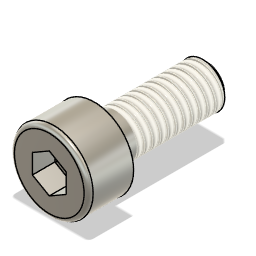
EchoWeather_WindVane (Autodesk Fusion 360 archive; units mm, degrees)
design "Broached Hexagon Socket Head Cap Screw ASME B18.3.1M - M4x0.7 x 10 Steel Grade 2 Plain"
description: Broached Hexagon Socket Head Cap Screw ASME B18.3.1M - M4x0.7 x 10
part number: BSHCS ASME B18.3.1M - M4x0.7 x 10 Steel Grade 2 Plain
Autodesk Fusion 360 part; units mm, degrees
note: some values were not read from the file. Chosen so that the rebuilt part matches the saved one: which bodies a step acts on; how an offset face is resized. Set by a fixed rule: which sketch regions a step uses.
sketch "Sketch1" plane through (0, 0, 0) normal (0, 1, 0) x (1, 0, 0)
  line L0 (-2, 0) -> (-2, 10)
  line L1 (-2, 10) -> (0, 10)
  line L2 (0, 10) -> (0, -4)
  line L3 (-2, 0) -> (-3.5, 0)
  line L4 (-3.5, 0) -> (-3.5, -4)
  line L5 (-3.5, -4) -> (0, -4)
  dimension "d9" = 4
  dimension "d66" = 7
  dimension "d101" = 10
  dimension "d102" = 4
  constraint perpendicular L0 L1
  constraint collinear origin L1.end L2.end
  constraint perpendicular L0 L3
  constraint coincident origin L3
  constraint vertical L0
  constraint vertical L2
  constraint parallel L2 L4
  constraint coincident L2 L5.end
  constraint perpendicular L2 L5
  measures "d101" distance of origin L1
  measures "d102" distance of L3.end L5
revolve "Revolve1" add sketch "Sketch1" angle 360 about axis through (0, 0, -10) along (0, 0, 1)
ref_plane "WorkPlane1" through (0, 0, 4) normal (0, 0, 1) x (1, 0, 0)
sketch "Sketch6" plane through (0, 0, 4) normal (0, 0, 1) x (1, 0, 0)
  line L0 (-1.5, 0) -> (1.5, 0) construction
  line L1 (0, 0) -> (-1.5, 0.866)
  line L2 (-1.5, -0.866) -> (-1.5, 0.866)
  line L3 (-1.5, -0.866) -> (0, 0)
  dimension "d100" = 150
  dimension "d103" = 3
  constraint horizontal L0
  constraint midpoint L1.start L0
  constraint coincident L1.start L3.end
  constraint perpendicular L0 L2
  constraint midpoint L0.start L2
  constraint coincident L1.end L2.end
  measures "d100" angle of L0 L1
  measures "d103" distance of L0.end L2
extrude "Extrude1" cut sketch "Sketch6" against normal blind 2
pattern_circular "C-Pattern1" count 6 over 360 about axis through (0, 0, 1.75) along (0, 0, 1) of "Extrude1"
extrude "Extrude2" cut 1 faces at (0, -0.5774, 2) along direction (0, 0, -1) blind 2 draft -85
thread "Thread3" "ANSI Metric M Profile 4.0 M4x0.7 M4x0.7 4g6g" major diameter 3.908 minor diameter 3.128 pitch 0.7 angle 60 resizes the face on face at (-1.9901, 0.1991, -3.3333)
fillet "Fillet4" radius 0.4 1 edges at (-3.2631, 1.2657, 4)
sketch "Sketch7" plane through (0, 0, 0) normal (0, 1, 0) x (1, 0, 0)
  line L0 (-2.04, 10) -> (-2.04, 9.5706)
  line L1 (-2.04, 9.5706) -> (-1.5706, 10)
  line L2 (0, 10) -> (0, -4)
  line L3 (-2.04, 10) -> (0, 10)
  dimension "d104" = 1.5706
  dimension "d105" = 2.04
  dimension "d106" = 0.4294
  constraint coincident L2.start L3.end
  constraint perpendicular L2 L3
  constraint coincident L1.end L3
  constraint perpendicular L0 L3
  measures "d104" distance of L1.end L2
  measures "d105" distance of L0 L2.start
  measures "d106" distance of L0.end L3
revolve "Revolve3" cut sketch "Sketch7" angle 360 about axis through (0, 0, 1.75) along (0, 0, 1)
equation "d9 = adsk_nomdia"
equation "adsk_nomlen = 10.00 mm"
equation "adsk_headh = 4.00 mm"
equation "adsk_headdia = 7.00 mm"
equation "adsk_nomdia = 4.00 mm"
equation "adsk_philwidth = 3.00 mm"
equation "d31 = -adsk_phildepth"
equation "adsk_phildepth = 2.00 mm"
equation "d66 = adsk_headdia"
equation "d71 = adsk_headh"
equation "d76 = -adsk_phildepth"
equation "adsk_thrlen = 8.170585 mm"
equation "d86 = adsk_nomdia * 0.1"
equation "adsk_startlen = 0.429415 mm"
equation "adsk_endpointdia = 3.14117 mm"
equation "d101 = adsk_nomlen"
equation "d102 = adsk_headh"
equation "d103 = adsk_philwidth"
equation "d104 = adsk_endpointdia / 2"
equation "d105 = adsk_nomdia * 0.51"
equation "d106 = adsk_startlen"
equation "d108 = min(adsk_thrlen; adsk_nomlen - 0.001 mm)"

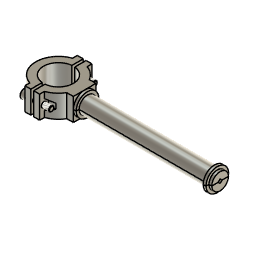
design "EchoWeather_SupportRod" references "Broached Hexagon Socket Head Cap Screw ASME B18.3.1M - M6x1 x 25 Steel Grade 2 Plain"
Autodesk Fusion 360 part; units mm, degrees
sketch "Sketch1" plane through (0, 0, 0) normal (0, 0, 1) x (1, 0, 0)
  circle A0 centre (0, 0) radius 16.764
  circle A1 centre (0, 0) radius 25.4
  dimension "d1" = 33.528
  dimension "d2" = 50.8
  constraint coincident A0.centre A1.centre
  measures "d1" diameter of A0
  measures "d2" diameter of A1
extrude "Extrude1" add sketch "Sketch1" along normal blind 25.4 makes body 1
sketch "Sketch2" plane through (0, 0, 0) normal (1, 0, 0) x (0, 1, 0)
  line L0 (0, 0) -> (0, 25.4) construction
  line L1 (25.4, 25.4) -> (-25.4, 25.4) construction
  circle A0 centre (0, 12.7) radius 9.525 construction
  line L2 (-12.7, 25.4) -> (12.7, 25.4)
  line L3 (12.7, 25.4) -> (12.7, 0)
  line L4 (12.7, 0) -> (-12.7, 0)
  line L5 (-12.7, 0) -> (-12.7, 25.4)
  line L6 (25.4, 0) -> (-25.4, 0)
  circle A1 centre (0, 12.7) radius 9.779
  dimension "d5" = 19.05
  dimension "d6" = 12.7
  dimension "d7" = 12.7
  dimension "d8" = 0.254
  constraint coincident L0.start origin
  constraint vertical L0
  constraint midpoint L0.end L1
  constraint midpoint L0 A0.centre
  constraint horizontal L2
  constraint vertical L3
  constraint horizontal L4
  constraint vertical L5
  constraint coincident L1 L2.start
  constraint coincident L3.end L6
  constraint concentric A0 A1
  measures "d5" diameter of A0
  measures "d6" distance of L0 L5
  measures "d7" distance of L0 L3
  measures "d8" distance of A0 A1
extrude "Extrude2" cut sketch "Sketch2" along normal blind 39.6494 contours A1 bodies 1
extrude "Extrude3" add sketch "Sketch2" along normal blind 12.7 from surface at 16.764 bodies 1
sketch "Sketch3" plane through (0, 0, 25.4) normal (0, 0, 1) x (-1, 0, 0)
  arc A0 (-21.997, -12.7) -> (-21.997, 12.7) centre (0, 0) ccw
  line L0 (-21.997, 12.7) -> (-29.464, 12.7)
  line L1 (-29.464, 12.7) -> (-29.464, -12.7)
  line L2 (-29.464, -12.7) -> (-21.997, -12.7)
  circle A1 centre (0, 0) radius 16.764
  line L3 (0, 0) -> (0, 34.343) construction
  line L4 (-8.255, 29.464) -> (8.255, 29.464)
  line L5 (8.255, 29.464) -> (8.255, 16.764)
  line L6 (8.255, 16.764) -> (-8.255, 16.764)
  line L7 (-8.255, 16.764) -> (-8.255, 29.464)
  line L8 (0, 0) -> (42.1929, 0) construction
  line L9 (8.255, -29.464) -> (8.255, -16.764)
  line L10 (-8.255, -16.764) -> (-8.255, -29.464)
  line L11 (-8.255, -29.464) -> (8.255, -29.464)
  line L12 (8.255, -16.764) -> (-8.255, -16.764)
  point P0 (0, -34.343)
  dimension "d14" = 12.7
  dimension "d15" = 8.255
  constraint coincident A0.centre A1.centre
  constraint parallel L1 L3
  constraint horizontal L4
  constraint vertical L5
  constraint horizontal L6
  constraint vertical L7
  constraint symmetric L3 L5 L7
  constraint tangent A1 L6
  constraint perpendicular L3 L8
  constraint symmetric L3.end L8 P0
  constraint symmetric L4.start L8 L10.end
  constraint symmetric L4.end L8 L9.start
  constraint symmetric L5.end L8 L9.end
  constraint symmetric L6.end L8 L10.start
  measures "d14" distance of L4 L6
  measures "d15" distance of L3 L5
extrude "Extrude4" add sketch "Sketch3" against normal up to surface (25.4 mm away) contours A0 L9 L10 L11 | A0 L4 L5 L7 bodies 1
sketch "Sketch4" plane through (-8.255, 0, 0) normal (-1, 0, 0) x (0, -1, 0)
  line L0 (-29.464, 0) -> (-24.0211, 0)
  line L1 (-24.0211, 0) -> (-24.0211, 25.4)
  line L2 (-24.0211, 25.4) -> (-29.464, 25.4)
  line L3 (-29.464, 25.4) -> (-29.464, 0)
  line L4 (-29.464, 12.7) -> (29.464, 12.7) construction
  line L5 (29.464, 25.4) -> (29.464, 0) construction
  circle A0 centre (-24.384, 12.7) radius 3.1
  circle A1 centre (24.384, 12.7) radius 3.1
  dimension "d18" = 6.2
  dimension "d19" = 6.2
  dimension "d20" = 5.08
  dimension "d21" = 5.08
  constraint midpoint L3 L4.start
  constraint perpendicular L1 L4
  constraint coincident L4.end L5
  constraint coincident L4 A0.centre
  constraint coincident L4 A1.centre
  measures "d18" diameter of A1
  measures "d19" diameter of A0
  measures "d20" distance of L3 A0.centre
  measures "d21" distance of L5 A1.centre
extrude "Extrude5" cut sketch "Sketch4" along normal blind 19.685 and the other way blind 31.4452 contours L1 A0 | L1 A0 | A1 bodies 1
sketch "Sketch5" plane through (-8.255, 0, 0) normal (-1, 0, 0) x (0, -1, 0)
  arc A0 (-24.0211, 15.7787) -> (-24.0211, 9.6213) centre (-24.384, 12.7) ccw
  line L0 (-24.0211, 15.7787) -> (-24.0211, 25.4)
  line L1 (-24.0211, 25.4) -> (-29.464, 25.4)
  line L2 (-29.464, 25.4) -> (-29.464, 0)
  line L3 (-29.464, 0) -> (-24.0211, 0)
  line L4 (-24.0211, 0) -> (-24.0211, 9.6213)
  circle A1 centre (-24.384, 12.7) radius 5.08
  arc A2 (24.0211, 9.6213) -> (24.0211, 15.7787) centre (24.384, 12.7) ccw construction
  circle A3 centre (24.384, 12.7) radius 5.08
  dimension "d26" = 10.16
  constraint concentric A0 A1
  constraint concentric A2 A3
  constraint equal A1 A3
  measures "d26" diameter of A1
extrude "Extrude6" cut sketch "Sketch5" along normal blind 27.3304 contours A0 L0 L4 A1 | A0 L0 L4 A1 | A3 bodies 1
sketch "Sketch6" plane through (8.255, 0, 0) normal (1, 0, 0) x (0, 1, 0)
  arc A0 (24.0211, 9.6213) -> (24.0211, 15.7787) centre (24.384, 12.7) ccw
  line L0 (24.0211, 9.6213) -> (24.0211, 0)
  line L1 (24.0211, 0) -> (29.464, 0)
  line L2 (29.464, 0) -> (29.464, 25.4)
  line L3 (29.464, 25.4) -> (24.0211, 25.4)
  line L4 (24.0211, 25.4) -> (24.0211, 15.7787)
  line L5 (24.384, 18.5659) -> (19.304, 15.6329)
  line L6 (19.304, 15.6329) -> (19.304, 9.7671)
  line L7 (19.304, 9.7671) -> (24.384, 6.8341)
  line L8 (24.384, 6.8341) -> (29.464, 9.7671)
  line L9 (29.464, 9.7671) -> (29.464, 15.6329)
  line L10 (29.464, 15.6329) -> (24.384, 18.5659)
  line L11 (0, 0) -> (0, 34.6531) construction
  line L12 (-24.384, 6.8341) -> (-29.464, 9.7671)
  line L13 (-24.384, 18.5659) -> (-19.304, 15.6329)
  line L14 (-29.464, 9.7671) -> (-29.464, 15.6329)
  line L15 (-19.304, 15.6329) -> (-19.304, 9.7671)
  line L16 (-19.304, 9.7671) -> (-24.384, 6.8341)
  line L17 (-29.464, 15.6329) -> (-24.384, 18.5659)
  arc A1 (-24.0211, 15.7787) -> (-24.0211, 9.6213) centre (-24.384, 12.7) ccw
  point P0 (24.384, 12.7)
  point P1 (-24.384, 12.7)
  dimension "d29" = 10.16
  constraint coincident P0 A0.centre
  constraint coincident L2 L9.end
  constraint coincident L11.start origin
  constraint vertical L11
  constraint symmetric A0.start L11 A1.end
  constraint symmetric A0.end L11 A1.start
  constraint symmetric A0 L11 A1
  constraint symmetric L5.start L11 L13.start
  constraint symmetric L5.end L11 L13.end
  constraint symmetric L6.end L11 L15.end
  constraint symmetric L7.end L11 L12.start
  constraint symmetric L8.end L11 L12.end
  constraint symmetric L9.end L11 L14.end
  constraint symmetric P0 L11 P1
  measures "d29" distance of L6 L9
extrude "Extrude7" cut sketch "Sketch6" along normal blind 15.0622 contours A0 L0 L4 L5 L6 L7 | A0 L0 L2 L4 L5 L7 L8 L9 L10 | L12 L13 L14 L15 L16 L17 bodies 1
sketch "Sketch7" plane through (0, 0, 25.4) normal (0, 0, 1) x (-1, 0, 0)
  arc A0 (-21.997, -12.7) -> (-8.255, -24.0211) centre (0, 0) ccw
  line L0 (-8.255, -24.0211) -> (-8.255, -29.464)
  line L1 (-8.255, -29.464) -> (8.255, -29.464)
  line L2 (8.255, -29.464) -> (8.255, -24.0211)
  arc A1 (8.255, -24.0211) -> (8.255, 24.0211) centre (0, 0) ccw
  line L3 (8.255, 24.0211) -> (8.255, 29.464)
  line L4 (8.255, 29.464) -> (-8.255, 29.464)
  line L5 (-8.255, 29.464) -> (-8.255, 24.0211)
  arc A2 (-8.255, 24.0211) -> (-21.997, 12.7) centre (0, 0) ccw
  line L6 (-21.997, 12.7) -> (-29.464, 12.7)
  line L7 (-29.464, 12.7) -> (-29.464, -12.7)
  line L8 (-29.464, -12.7) -> (-21.997, -12.7)
  circle A3 centre (0, 0) radius 16.764
  line L9 (-1.5875, 29.464) -> (1.5875, 29.464)
  line L10 (1.5875, 29.464) -> (1.5875, -29.464)
  line L11 (1.5875, -29.464) -> (-1.5875, -29.464)
  line L12 (-1.5875, -29.464) -> (-1.5875, 29.464)
  line L13 (0, -29.464) -> (0, 29.464) construction
  dimension "d32" = 1.5875
  constraint horizontal L9
  constraint vertical L10
  constraint horizontal L11
  constraint vertical L12
  constraint coincident L1 L10.end
  constraint coincident L4 L9.start
  constraint midpoint L11 L13.start
  constraint midpoint L9 L13.end
  constraint coincident A0.centre L13
  measures "d32" distance of L10 L13
extrude "Extrude8" cut sketch "Sketch7" against normal blind 35.1536 contours L1 A3 L10 L11 L12 | L4 A3 L9 L10 L12 bodies 1 makes body 2 at (3.2193, -16.452, 8.4667)
sketch "Sketch8" plane through (29.464, 0, 0) normal (1, 0, 0) x (0, 1, 0)
  circle A0 centre (0, 12.7) radius 9.779
  line L0 (12.7, 25.4) -> (-12.7, 25.4)
  line L1 (-12.7, 25.4) -> (-12.7, 0)
  line L2 (-12.7, 0) -> (12.7, 0)
  line L3 (12.7, 0) -> (12.7, 25.4)
  line L4 (0, 0) -> (0, 25.4) construction
  line L5 (0, 12.7) -> (31.6085, 12.7) construction
  circle A1 centre (0, 12.7) radius 9.398
  circle A2 centre (0, 12.7) radius 12.7
  dimension "d35" = 18.796
  dimension "d36" = 25.4
  constraint coincident L4.start origin
  constraint midpoint L0 L4.end
  constraint coincident A0.centre L5.start
  constraint perpendicular L4 L5
  measures "d35" diameter of A1
  measures "d36" diameter of A2
extrude "Extrude9" add sketch "Sketch8" along normal blind 152.4 and the other way blind 12.7 separate body contours A1 makes body 3
extrude "Extrude10" add sketch "Sketch8" along normal blind 3.175 contours A0 | A2 bodies 3
sketch "Sketch10" plane through (181.864, 0, 0) normal (1, 0, 0) x (0, 1, 0)
  circle A0 centre (0, 12.7) radius 9.398
  circle A1 centre (0, 12.7) radius 12.7
  dimension "d43" = 25.4
  constraint concentric A0 A1
  measures "d43" diameter of A1
extrude "Extrude11" add sketch "Sketch10" against normal blind 3.175 from surface at -3.175 bodies 3
sketch "Sketch11" plane through (181.864, 0, 0) normal (1, 0, 0) x (0, 1, 0)
  circle A0 centre (0, 12.7) radius 9.398
  line L0 (0, 12.7) -> (35.7473, 12.7) construction
  line L1 (0, 12.7) -> (0, 36.2034) construction
  line L2 (0, 14.9451) -> (2.2451, 12.7)
  line L3 (2.2451, 12.7) -> (0, 10.4549)
  line L4 (0, 10.4549) -> (-2.2451, 12.7)
  line L5 (-2.2451, 12.7) -> (0, 14.9451)
  dimension "d58" = 45
  dimension "d59" = 3.175
  constraint coincident A0.centre L0.start
  constraint horizontal L0
  constraint perpendicular L0 L1
  constraint perpendicular L2 L3
  constraint parallel L2 L4
  constraint parallel L3 L5
  constraint coincident L1 L2.start
  constraint coincident L0 L2.end
  constraint equal L2 L3
  measures "d58" angle of L0 L2
  measures "d59" distance of L2 L4
extrude "Extrude12" cut sketch "Sketch11" against normal up to surface (165.1 mm away) contours L2 L3 L4 L5 bodies 3
ref_plane "WorkPlane1" through (15.5258, 0, 12.7) normal (0, 0, 1) x (1, 0, 0)
split "Split1" by plane through (15.5258, 0, 12.7) normal (0, 0, 1) bodies 3 makes body 4 at (127.889, 8.2535, 17.1946)
other "Screw1"
other "Screw2"
component "EchoWeather_SupportRod v5" placed x (1, 0, 0) y (0, 1, 0) z (0, 0, 1) at (0, 0, 0)
component "EchoWeather_SupportRod v5" placed x (1, 0, 0) y (0, 1, 0) z (0, 0, 1) at (0, 0, 0)
named bodies: "OuterClamp", "Inner Clamp", "SupportA", "SupportB"

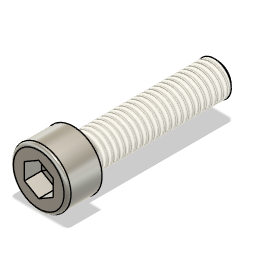
design "Broached Hexagon Socket Head Cap Screw ASME B18.3.1M - M6x1 x 25 Steel Grade 2 Plain"
description: Broached Hexagon Socket Head Cap Screw ASME B18.3.1M - M6x1 x 25
part number: BSHCS ASME B18.3.1M - M6x1 x 25 Steel Grade 2 Plain
Autodesk Fusion 360 part; units mm, degrees
sketch "Sketch1" plane through (0, 0, 0) normal (0, 1, 0) x (1, 0, 0)
  line L0 (-3, 0) -> (-3, 25)
  line L1 (-3, 25) -> (0, 25)
  line L2 (0, 25) -> (0, -6)
  line L3 (-3, 0) -> (-5, 0)
  line L4 (-5, 0) -> (-5, -6)
  line L5 (-5, -6) -> (0, -6)
  dimension "d9" = 6
  dimension "d66" = 10
  dimension "d101" = 25
  dimension "d102" = 6
  constraint perpendicular L0 L1
  constraint collinear origin L1.end L2.end
  constraint perpendicular L0 L3
  constraint coincident origin L3
  constraint vertical L0
  constraint vertical L2
  constraint parallel L2 L4
  constraint coincident L2 L5.end
  constraint perpendicular L2 L5
  measures "d101" distance of origin L1
  measures "d102" distance of L3.end L5
revolve "Revolve1" add sketch "Sketch1" angle 360 about axis through (0, 0, -25) along (0, 0, 1)
ref_plane "WorkPlane1" through (0, 0, 6) normal (0, 0, 1) x (1, 0, 0)
sketch "Sketch6" plane through (0, 0, 6) normal (0, 0, 1) x (1, 0, 0)
  line L0 (-2.5, 0) -> (2.5, 0) construction
  line L1 (0, 0) -> (-2.5, 1.4434)
  line L2 (-2.5, -1.4434) -> (-2.5, 1.4434)
  line L3 (-2.5, -1.4434) -> (0, 0)
  dimension "d100" = 150
  dimension "d103" = 5
  constraint horizontal L0
  constraint midpoint L1.start L0
  constraint coincident L1.start L3.end
  constraint perpendicular L0 L2
  constraint midpoint L0.start L2
  constraint coincident L1.end L2.end
  measures "d100" angle of L0 L1
  measures "d103" distance of L0.end L2
extrude "Extrude1" cut sketch "Sketch6" against normal blind 3
pattern_circular "C-Pattern1" count 6 over 360 about axis through (0, 0, 1.75) along (0, 0, 1) of "Extrude1"
extrude "Extrude2" cut 1 faces at (0.8333, -0.4811, 3) along direction (0, 0, -1) blind 3 draft -85
thread "Thread3" "ANSI Metric M Profile 6.0 M6x1 M6x1 4g6g" major diameter 5.884 minor diameter 4.764 pitch 1 angle 60 resizes the face on face at (-2.9963, 0.1495, -8.3333)
fillet "Fillet4" radius 0.6 1 edges at (-4.6616, 1.8081, 6)
sketch "Sketch7" plane through (0, 0, 0) normal (0, 1, 0) x (1, 0, 0)
  line L0 (-3.06, 25) -> (-3.06, 24.3866)
  line L1 (-3.06, 24.3866) -> (-2.3866, 25)
  line L2 (0, 25) -> (0, -6)
  line L3 (-3.06, 25) -> (0, 25)
  dimension "d104" = 2.3866
  dimension "d105" = 3.06
  dimension "d106" = 0.6135
  constraint coincident L2.start L3.end
  constraint perpendicular L2 L3
  constraint coincident L1.end L3
  constraint perpendicular L0 L3
  measures "d104" distance of L1.end L2
  measures "d105" distance of L0 L2.start
  measures "d106" distance of L0.end L3
revolve "Revolve3" cut sketch "Sketch7" angle 360 about axis through (0, 0, 1.75) along (0, 0, 1)
equation "d9 = adsk_nomdia"
equation "adsk_nomlen = 25.00 mm"
equation "adsk_headh = 6.00 mm"
equation "adsk_headdia = 10.00 mm"
equation "adsk_nomdia = 6.00 mm"
equation "adsk_philwidth = 5.00 mm"
equation "d31 = -adsk_phildepth"
equation "adsk_phildepth = 3.00 mm"
equation "d66 = adsk_headdia"
equation "d71 = adsk_headh"
equation "d76 = -adsk_phildepth"
equation "adsk_thrlen = 23.1731 mm"
equation "d86 = adsk_nomdia * 0.1"
equation "adsk_startlen = 0.61345 mm"
equation "adsk_endpointdia = 4.7731 mm"
equation "d101 = adsk_nomlen"
equation "d102 = adsk_headh"
equation "d103 = adsk_philwidth"
equation "d104 = adsk_endpointdia / 2"
equation "d105 = adsk_nomdia * 0.51"
equation "d106 = adsk_startlen"
equation "d108 = min(adsk_thrlen; adsk_nomlen - 0.001 mm)"
